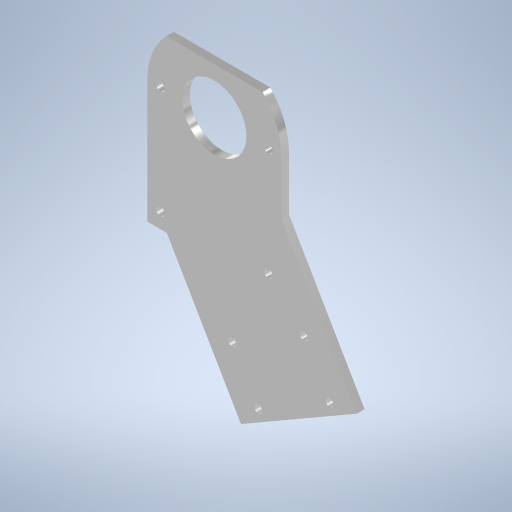
# Autodesk Inventor part: elbow
Saved by Autodesk Inventor 2024.1 (Build 281209000, 209)
## iProperties
Created: 2024-02-14
Part Number: elbow
Material: アルミニウム 6061
Document SubType Name: Modeling
Designer: hibik
Density: 2.7 g/cm^3
Appearance: アルミニウム - フラット
Author: hibik
Autodesk Inventor part; units mm, degrees
ref_plane "YZ Plane" through (0, 0, 0) normal (1, 0, 0) x (0, 1, 0)
ref_plane "XZ Plane" through (0, 0, 0) normal (0, 1, 0) x (-1, 0, 0)
ref_plane "XY Plane" through (0, 0, 0) normal (0, 0, 1) x (1, 0, 0)
sketch "スケッチ2" plane through (0, 0, 0) normal (0, 0, 1) x (1, 0, 0)
  line L0 (0, 0) -> (26, 0)
  line L1 (26, 0) -> (26, 33)
  line L2 (26, 33) -> (0, 33)
  line L3 (0, 33) -> (0, 0)
  line L4 (0, 0) -> (26, 0)
  line L5 (26, 0) -> (26, 24)
  line L6 (26, 24) -> (0, 24) construction
  line L7 (0, 24) -> (0, 0)
  circle A0 centre (13, 24) radius 13
  circle A1 centre (13, 24) radius 6.25
  line L8 (26, 0) -> (0, 0)
  line L9 (17.9352, 27.452) -> (40.6962, -11.9711)
  line L10 (40.6962, -11.9711) -> (18.1795, -24.9711)
  line L11 (18.1795, -24.9711) -> (-4.3205, 14)
  circle A2 centre (21.5096, -20.7391) radius 0.8
  circle A3 centre (35.366, -12.7391) radius 0.8
  line L12 (-4.3205, 14) -> (18.1962, 27)
  point P0 (22.3808, 33)
  point P1 (3.6192, 33)
  point P2 (26, 13.4833)
  point P3 (3.7624, 0)
  point P4 (23.9624, 17.0125)
  point P5 (1.7417, 17.5)
  point P6 (0, 16.4944)
  point P7 (0, 6.5167)
  point P8 (7.5873, 20.875)
  point P9 (19.0712, 25.4845)
  dimension "d0" = 26
  dimension "d1" = 33
  dimension "d2" = 24
  dimension "d3" = 12.5
  dimension "d14" = 26
  dimension "d17" = 1.6
  dimension "d18" = 1.6
  dimension "d19" = 2
  dimension "d20" = 2
  dimension "d21" = 5
  dimension "d22" = 5
  dimension "d23" = 20
  dimension "d25" = 45
  dimension "d26" = 30
  constraints: 26 end point, 5 parallel, 3 centre point, 3 horizontal, 3 perpendicular, 3 point on line, 1 coincident, 1 midpoint, 3 other
  measures "d0" distance of L1.end L2.end
  measures "d1" distance of L2.end L0.start
  measures "d2" distance between parallel lines of L0 L6
  measures "d3" diameter of A1
  measures "d14" distance between parallel lines of L11 L9
  measures "d17" diameter of A2
  measures "d18" diameter of A3
  measures "d19" distance from line of A2.centre L10
  measures "d20" distance from line of L10 A3.centre
  measures "d21" distance from line of L11 A2.centre
  measures "d22" distance from line of L9 A3.centre
  measures "d23" distance from line of L11 A1.centre
  measures "d25" distance between parallel lines of L10 L12
  measures "d26" angle of L9 L1
extrude "押し出し1" add sketch "スケッチ2" along normal blind 1.5 contours L3 L11 L0 | L11 L3 L12 A0 L9 L1 L0 | L0 L1 L9 L10 L11 | L3 A0 L12 | L9 A0 L1 | A0 L2 L9 A1 L12 | L12 A1 L9 A0
sketch "スケッチ3" plane through (0, 0, 0) normal (0, 0, -1) x (-1, 0, 0)
  circle A0 centre (-2.5, 24) radius 0.85 projected
  circle A1 centre (-23.5, 24) radius 0.85 projected
  circle A2 centre (-23.5, 3) radius 0.85 projected
  circle A3 centre (-2.5, 3) radius 0.85 projected
  circle A4 centre (-30.366, -4.0788) radius 0.8 projected
  circle A5 centre (-16.5096, -12.0788) radius 0.8 projected
  point P0 (0, 0)
extrude "押し出し2" cut sketch "スケッチ3" against normal through all
equation "\"d20\" = d19"
